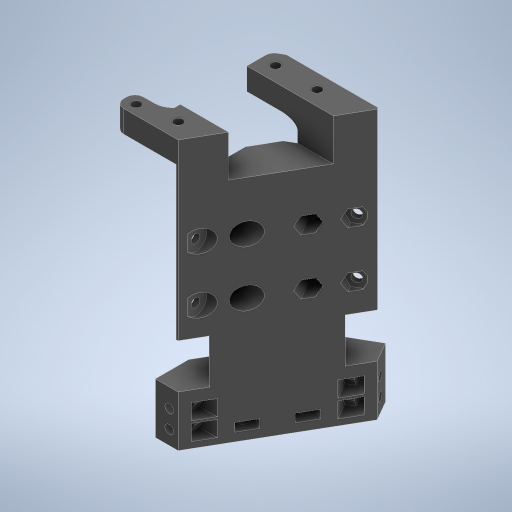
# Autodesk Inventor part: base_plate_towheel_front_right
Saved by Autodesk Inventor 2024.1 (Build 281209000, 209)
## iProperties
Created: 2025-02-03
Part Number: base_plate_towheel_front_right
Material: 一般
Document SubType Name: モデリング
Designer: hibik
Density: 1 g/cm^3
Appearance: 既定
Sheet Metal Rule: Default_mm
Author: hibik
Autodesk Inventor part; units mm, degrees
ref_plane "YZ Plane" through (0, 0, 0) normal (1, 0, 0) x (0, 1, 0)
ref_plane "XZ Plane" through (0, 0, 0) normal (0, 1, 0) x (-1, 0, 0)
ref_plane "XY Plane" through (0, 0, 0) normal (0, 0, 1) x (1, 0, 0)
sketch "スケッチ1" plane through (0, 0, 0) normal (0, 1, 0) x (-1, 0, 0)
  line L0 (75, 0) -> (105, -51.9615)
  line L1 (-75, 0) -> (-105, -51.9615)
  line L2 (0, -220.136) -> (0, 47.7586) projected
  line L3 (147, 0) -> (-147, 0) projected
  line L4 (37.5, -27) -> (-37.5, -27)
  line L5 (105, -51.9615) -> (30, -181.8653)
  line L6 (30, -181.8653) -> (-30, -181.8653)
  line L7 (-30, -181.8653) -> (-105, -51.9615)
  line L8 (75, 0) -> (-75, 0)
  line L9 (-25.3673, -135.8894) -> (-62.8673, -70.9375)
  line L10 (25.3673, -135.8894) -> (62.8673, -70.9375)
  line L11 (-37.5, -27) -> (-27.5, -27)
  line L12 (-27.5, -27) -> (-27.5, -39)
  line L13 (-27.5, -39) -> (-37.5, -39)
  line L14 (-37.5, -39) -> (-37.5, -27)
  line L15 (37.5, -27) -> (27.5, -27)
  line L16 (27.5, -27) -> (27.5, -39)
  line L17 (27.5, -39) -> (37.5, -39)
  line L18 (37.5, -39) -> (37.5, -27)
  line L19 (0, -77.9423) -> (44.1173, -103.4134) construction
  line L20 (0, -77.9423) -> (-44.1173, -103.4134) construction
  line L21 (-44.1173, -103.4134) -> (-67.5, -116.9134) construction
  line L22 (-57.8673, -79.5977) -> (-47.475, -73.5977)
  line L23 (-52.475, -64.9375) -> (-62.8673, -70.9375)
  line L24 (-62.8673, -70.9375) -> (-57.8673, -79.5977)
  line L25 (-47.475, -73.5977) -> (-52.475, -64.9375)
  line L26 (-25.3673, -135.8894) -> (-30.3673, -127.2291)
  line L27 (-19.975, -121.2291) -> (-14.975, -129.8894)
  line L28 (-14.975, -129.8894) -> (-25.3673, -135.8894)
  line L29 (-30.3673, -127.2291) -> (-19.975, -121.2291)
  line L30 (30.3673, -127.2291) -> (19.975, -121.2291)
  line L31 (14.975, -129.8894) -> (25.3673, -135.8894)
  line L32 (25.3673, -135.8894) -> (30.3673, -127.2291)
  line L33 (19.975, -121.2291) -> (14.975, -129.8894)
  line L34 (62.8673, -70.9375) -> (57.8673, -79.5977)
  line L35 (47.475, -73.5977) -> (52.475, -64.9375)
  line L36 (52.475, -64.9375) -> (62.8673, -70.9375)
  line L37 (57.8673, -79.5977) -> (47.475, -73.5977)
  line L38 (62.8673, -70.9375) -> (37.5, -27)
  line L39 (-37.5, -27) -> (-62.8673, -70.9375)
  line L40 (-25.3673, -135.8894) -> (25.3673, -135.8894)
  line L41 (-27.5, -39) -> (-47.475, -73.5977)
  point P0 (0, 0)
  point P1 (0, 0)
  point P2 (0, -27)
  dimension "d1" = 150
  dimension "d2" = 60
  dimension "d3" = 60
  dimension "d4" = 27
  dimension "d5" = 75
  dimension "d6" = 60
  dimension "d7" = 27
  dimension "d8" = 10
  dimension "d9" = 12
  dimension "d10" = 10
  dimension "d11" = 12
  dimension "d14" = 360
  constraints: 80 end point, 6 equal length, 6 parallel, 4 horizontal, 4 midpoint, 3 coincident, 3 perpendicular, 2 symmetric about line, 1 collinear, 1 horizontal alignment, 1 point on line, 1 vertical alignment, 50 other
  measures "d1" distance of L1.start L0.start
  measures "d2" angle of L3 L0
  measures "d3" angle of L1 L3
  measures "d4" distance between parallel lines of L3 L4
  measures "d5" distance of L4.start L4.end
  measures "d6" distance of L5.end L6.end
  measures "d7" distance between parallel lines of L7 L9
  measures "d8" distance of L12.end L13.end
  measures "d9" distance of L11.end L12.end
  measures "d10" distance of L17.end L16.end
  measures "d11" distance of L16.end L15.end
extrude "押し出し1" add sketch "スケッチ1" along normal blind 18.3 contours L12 L13 L14 L4 | L14 L13 L41 L25 L23 L39 | L23 L25 L22 L9
sketch "スケッチ2" plane through (27.5, 0, -27) normal (0, 0, 1) x (1, 0, 0)
  circle A0 centre (5, 11.5) radius 1.6 projected
  circle A1 centre (5, 5) radius 1.6 projected
  point P0 (-27.5, 0)
sketch "スケッチ3" plane through (27.5, 0, -27) normal (0, 0, 1) x (1, 0, 0)
  circle A0 centre (5, 11.5) radius 1.6 projected
  circle A1 centre (5, 5) radius 1.6 projected
  line L0 (8.2909, 11.5) -> (6.6454, 8.65)
  line L1 (6.6454, 8.65) -> (3.3546, 8.65)
  line L2 (3.3546, 8.65) -> (1.7091, 11.5)
  line L3 (1.7091, 11.5) -> (3.3546, 14.35)
  line L4 (3.3546, 14.35) -> (6.6454, 14.35)
  line L5 (6.6454, 14.35) -> (8.2909, 11.5)
  line L6 (6.6454, 7.85) -> (8.2909, 5)
  line L7 (8.2909, 5) -> (6.6454, 2.15)
  line L8 (6.6454, 2.15) -> (3.3546, 2.15)
  line L9 (3.3546, 2.15) -> (1.7091, 5)
  line L10 (1.7091, 5) -> (3.3546, 7.85)
  line L11 (3.3546, 7.85) -> (6.6454, 7.85)
  point P0 (-27.5, 0)
  dimension "d19" = 5.7
  constraints: 24 end point, 2 coincident, 2 horizontal, 1 parallel, 26 other
  measures "d19" distance from line of L0.end L4
extrude "押し出し2" cut sketch "スケッチ3" against normal blind 6 contours A0 | A1 | L0 L1 L2 L3 L4 L5 | L6 L7 L8 L9 L10 L11
extrude "押し出し3" add sketch "スケッチ3" against normal blind 3
sketch "スケッチ4" plane through (27.5, 0, -33) normal (0, 0, 1) x (1, 0, 0)
  line L0 (3.3546, 14.35) -> (6.6454, 14.35)
  line L1 (1.7091, 11.5) -> (3.3546, 14.35)
  line L2 (3.3546, 8.65) -> (1.7091, 11.5)
  line L3 (6.6454, 8.65) -> (3.3546, 8.65)
  line L4 (1.7091, 5) -> (3.3546, 7.85)
  line L5 (3.3546, 2.15) -> (1.7091, 5)
  line L6 (6.6454, 2.15) -> (3.3546, 2.15)
  line L7 (3.3546, 7.85) -> (6.6454, 7.85)
  line L8 (3.3546, 14.35) -> (6.6454, 14.35) projected
  line L9 (6.6454, 14.35) -> (42.8044, 14.35)
  line L10 (42.8044, 14.35) -> (42.8044, 8.65)
  line L11 (42.8044, 8.65) -> (6.6454, 8.65)
  line L12 (6.6454, 7.85) -> (42.8044, 7.85)
  line L13 (42.8044, 7.85) -> (42.8044, 2.15)
  line L14 (42.8044, 2.15) -> (6.6454, 2.15)
  line L15 (6.6454, 14.35) -> (3.3546, 14.35) projected
  line L16 (3.3546, 14.35) -> (1.7091, 11.5) projected
  line L17 (1.7091, 11.5) -> (3.3546, 8.65) projected
  line L18 (3.3546, 8.65) -> (6.6454, 8.65) projected
  line L19 (3.3546, 7.85) -> (1.7091, 5) projected
  line L20 (6.6454, 7.85) -> (3.3546, 7.85) projected
  line L21 (8.2909, 5) -> (6.6454, 7.85) projected
  line L22 (6.6454, 2.15) -> (8.2909, 5) projected
  line L23 (3.3546, 2.15) -> (6.6454, 2.15) projected
  line L24 (1.7091, 5) -> (3.3546, 2.15) projected
  circle A0 centre (5, 5) radius 1.6 projected
  line L25 (6.6454, 7.85) -> (3.3546, 7.85) projected
  line L26 (3.3546, 7.85) -> (1.7091, 5) projected
  line L27 (1.7091, 5) -> (3.3546, 2.15) projected
  line L28 (3.3546, 2.15) -> (6.6454, 2.15) projected
  point P0 (-27.5, 0)
  constraints: 28 end point, 2 horizontal, 2 parallel, 2 perpendicular, 2 point on line, 1 collinear
extrude "押し出し4" cut sketch "スケッチ4" along normal blind 3 contours L0 L9 L10 L11 L3 L2 L1 | L4 L7 L21 L22 L6 L5 | L12 L13 L14 L22 L21 | A0
sketch "スケッチ5" plane through (62.8673, 0, -70.9375) normal (0.8660254, 0, 0.5) x (0.5, 0, -0.8660254)
  line L0 (-5.3923, 18.3) -> (-45.3423, 18.3) projected
  line L1 (-25.3673, 18.3) -> (-25.3673, 0)
  line L2 (-5.3923, 0) -> (-45.3423, 0) projected
  point P0 (-92.8673, 0)
  constraints: 2 end point, 2 midpoint
ref_plane "作業平面1" through (50.1837, 18.3, -48.9687) normal (-0.5, 0, 0.8660254) x (0, -1, 0)
mirror "ミラー1" about plane through (50.1837, 18.3, -48.9687) normal (-0.5, 0, 0.8660254) of "押し出し2", "押し出し3", "押し出し4"
sketch "スケッチ6" plane through (0, 0, 0) normal (0, -1, 0) x (1, 0, 0)
  line L0 (37.5, -27) -> (62.8673, -70.9375) projected
  circle A0 centre (40.9875, -45.0405) radius 1.6
  line L1 (42.7196, -48.0405) -> (39.2555, -48.0405)
  line L2 (39.2555, -48.0405) -> (37.5234, -45.0405)
  line L3 (37.5234, -45.0405) -> (39.2555, -42.0405)
  line L4 (39.2555, -42.0405) -> (42.7196, -42.0405)
  line L5 (42.7196, -42.0405) -> (44.4516, -45.0405)
  line L6 (44.4516, -45.0405) -> (42.7196, -48.0405)
  line L7 (50.1837, -48.9687) -> (37.4875, -56.2989)
  line L8 (47.475, -73.5977) -> (27.5, -39) projected
  line L9 (37.6966, -45.0405) -> (39.3421, -42.1905)
  line L10 (39.3421, -42.1905) -> (42.633, -42.1905)
  line L11 (42.633, -42.1905) -> (44.2784, -45.0405)
  line L12 (44.2784, -45.0405) -> (42.633, -47.8905)
  line L13 (42.633, -47.8905) -> (39.3421, -47.8905)
  line L14 (39.3421, -47.8905) -> (37.6966, -45.0405)
  point P0 (0, 0)
  dimension "d27" = 3.2
  dimension "d29" = 6
  dimension "d30" = 6
  dimension "d31" = 8
  dimension "d32" = 5.7
  constraints: 26 end point, 2 coincident, 2 midpoint, 2 parallel, 1 centre point, 26 other
  measures "d27" diameter of A0
  measures "d29" distance between parallel lines of L2 L5
  measures "d30" distance from line of L0 A0.centre
  measures "d31" distance from line of L7 A0.centre
  measures "d32" distance between parallel lines of L14 L11
extrude "押し出し5" cut sketch "スケッチ6" against normal through all contours A0 | L9 L10 L11 L12 L13 L14
extrude "押し出し7" add sketch "スケッチ6" against normal blind 3 contours L9 L10 L11 L12 L13 L14
mirror "ミラー2" about plane through (50.1837, 18.3, -48.9687) normal (-0.5, 0, 0.8660254) of "押し出し5", "押し出し7"
sketch "スケッチ10" plane through (0, 0, 0) normal (0, -1, 0) x (1, 0, 0)
  line L0 (75, 0) -> (105, -51.9615)
  line L1 (75, 0) -> (81.3804, 3.6837)
  line L2 (37.5, -27) -> (62.8673, -70.9375) projected
  line L3 (50.1837, -48.9687) -> (90, -25.9808)
  line L4 (-21, 0) -> (126, 0) projected
  line L5 (75, 0) -> (35, 0)
  line L6 (45, 0) -> (45, -18)
  line L7 (45, -18) -> (35, -23.7735)
  line L8 (35, 0) -> (35, -23.7735)
  line L9 (35, -23.7735) -> (49.7058, -49.2446)
  line L10 (105, -51.9615) -> (75, 0)
  line L11 (85, -86.6025) -> (64.4115, -74.7158)
  line L12 (64.4115, -74.7158) -> (49.7058, -49.2446)
  line L13 (85, -86.6025) -> (105, -51.9615)
  line L14 (62.8673, -70.9375) -> (57.8673, -79.5977) projected
  line L15 (61.9714, -72.4893) -> (35.6987, -26.9836)
  line L16 (27.5, -27) -> (37.5, -27) projected
  point P0 (0, 0)
  point P1 (35.7081, -27)
  dimension "d47" = 60
  dimension "d48" = 40
  dimension "d49" = 18
  dimension "d50" = 30
  dimension "d51" = 60
  dimension "d63" = 1
  constraints: 28 end point, 5 perpendicular, 5 point on line, 4 symmetric about line, 2 midpoint, 2 parallel
  measures "d47" distance from line of L0.end L1
  measures "d48" distance of L5.end L0.start
  measures "d49" distance of L6.start L6.end
  measures "d50" distance of L0.start L6.start
  measures "d51" angle of L6 L7
  measures "d63" distance between parallel lines of L12 L15
sketch "スケッチ8" plane through (0, 18.3, 0) normal (0, 1, 0) x (1, 0, 0)
  line L0 (47.475, 73.5977) -> (27.5, 39) projected
  line L1 (47.3421, 61.7469) -> (50.633, 61.7469) projected
  line L2 (50.633, 61.7469) -> (52.2784, 58.8969) projected
  line L3 (52.2784, 58.8969) -> (50.633, 56.0469) projected
  line L4 (50.633, 56.0469) -> (47.3421, 56.0469) projected
  line L5 (47.3421, 56.0469) -> (45.6966, 58.8969) projected
  line L6 (45.6966, 58.8969) -> (47.3421, 61.7469) projected
  line L7 (42.633, 47.8905) -> (44.2784, 45.0405) projected
  line L8 (44.2784, 45.0405) -> (42.633, 42.1905) projected
  line L9 (42.633, 42.1905) -> (39.3421, 42.1905) projected
  line L10 (39.3421, 42.1905) -> (37.6966, 45.0405) projected
  line L11 (37.6966, 45.0405) -> (39.3421, 47.8905) projected
  line L12 (39.3421, 47.8905) -> (42.633, 47.8905) projected
  line L13 (57.8673, 79.5977) -> (47.475, 73.5977) projected
  line L14 (47.475, 73.5977) -> (27.5, 39) projected
  line L15 (27.5, 39) -> (27.5, 27) projected
  line L16 (27.5, 27) -> (37.5, 27) projected
  line L17 (37.5, 27) -> (62.8673, 70.9375) projected
  line L18 (62.8673, 70.9375) -> (57.8673, 79.5977) projected
  line L19 (42.633, 47.8905) -> (47.8291, 44.8905)
  line L20 (39.3421, 42.1905) -> (44.5382, 39.1905)
  line L21 (47.3421, 56.0469) -> (52.5382, 53.0469)
  line L22 (50.633, 61.7469) -> (55.8291, 58.7469)
  line L23 (37.5, 27) -> (62.8673, 70.9375) projected
  point P0 (0, 0)
  constraints: 8 end point, 4 perpendicular, 4 point on line
extrude "押し出し9" cut sketch "スケッチ8" against normal up to surface (15.3 mm away) contours L17 L21 L4 L3 L2 L22 | L20 L9 L8 L7 L19 L17
sketch "スケッチ11" plane through (0, 18.3, 0) normal (0, 1, 0) x (1, 0, 0)
  line L0 (52.5382, 53.0469) -> (47.3421, 56.0469) projected
  line L1 (47.3421, 56.0469) -> (45.6966, 58.8969) projected
  line L2 (45.6966, 58.8969) -> (47.3421, 61.7469) projected
  line L3 (47.3421, 61.7469) -> (50.633, 61.7469) projected
  line L4 (50.633, 61.7469) -> (55.8291, 58.7469) projected
  line L5 (55.8291, 58.7469) -> (62.8673, 70.9375) projected
  line L6 (62.8673, 70.9375) -> (57.8673, 79.5977) projected
  line L7 (57.8673, 79.5977) -> (47.475, 73.5977) projected
  line L8 (47.475, 73.5977) -> (27.5, 39) projected
  line L9 (27.5, 39) -> (27.5, 27) projected
  line L10 (27.5, 27) -> (37.5, 27) projected
  line L11 (37.5, 27) -> (44.5382, 39.1905) projected
  line L12 (44.5382, 39.1905) -> (39.3421, 42.1905) projected
  line L13 (39.3421, 42.1905) -> (37.6966, 45.0405) projected
  line L14 (37.6966, 45.0405) -> (39.3421, 47.8905) projected
  line L15 (39.3421, 47.8905) -> (42.633, 47.8905) projected
  line L16 (42.633, 47.8905) -> (47.8291, 44.8905) projected
  line L17 (47.8291, 44.8905) -> (52.5382, 53.0469) projected
  line L18 (38.5, 27) -> (38.5, 38)
  line L19 (38.5, 38) -> (29.817, 43.0131)
  line L20 (27.5, 27) -> (37.5, 27) projected
  line L21 (47.475, 73.5977) -> (27.5, 39) projected
  line L22 (50.1837, 48.9687) -> (37.4875, 56.2989)
  line L23 (63.3673, 70.0715) -> (53.841, 64.5715)
  line L24 (53.841, 64.5715) -> (45.158, 69.5846)
  line L25 (47.8291, 44.8905) -> (44.5382, 39.1905) projected
  line L26 (55.8291, 58.7469) -> (52.5382, 53.0469) projected
  point P0 (0, 0)
  point P1 (61.8673, 69.2054)
  point P2 (38.5, 28.7321)
  dimension "d52" = 1
  dimension "d53" = 11
  constraints: 10 end point, 3 perpendicular, 3 symmetric about line, 2 midpoint, 2 point on line
  measures "d52" distance from line of L10.end L18
  measures "d53" distance of L18.start L18.end
extrude "押し出し11" add sketch "スケッチ11" along normal blind 78.7 contours L17 L22 L8 L24 L23 L5 L4 L3 L2 L1 L0 | L0 L1 L2 L3 L4 L26 | L17 L16 L15 L14 L13 L12 L11 L18 L19 L8 L22 | L25 L12 L13 L14 L15 L16
fillet "フィレット1" radius 2 2 edges at (38.5, 57.65, -28.7321) (61.8673, 57.65, -69.2054)
sketch "スケッチ13" plane through (0, 97, 0) normal (0, 1, 0) x (1, 0, 0)
  line L0 (85, 86.6025) -> (64.4115, 74.7158) projected
  line L1 (35, 0) -> (35, 23.7735) projected
  arc A0 (58.1353, 62.7413) -> (55.4032, 65.4734) centre (56.4032, 63.7413) ccw projected
  line L2 (55.4032, 65.4734) -> (53.841, 64.5715) projected
  line L3 (53.841, 64.5715) -> (45.158, 69.5846) projected
  line L4 (45.158, 69.5846) -> (29.817, 43.0131) projected
  line L5 (29.817, 43.0131) -> (38.5, 38) projected
  line L6 (38.5, 38) -> (38.5, 36.1962) projected
  arc A1 (38.5, 36.1962) -> (42.2321, 35.1962) centre (40.5, 36.1962) ccw projected
  line L7 (35, 23.7735) -> (35, 57.735)
  line L8 (35, 57.735) -> (64.4115, 74.7158)
  line L9 (38.5, 38) -> (29.817, 43.0131) projected
  line L10 (29.817, 43.0131) -> (27.5, 39) projected
  line L11 (27.5, 39) -> (27.5, 27) projected
  line L12 (27.5, 27) -> (37.5, 27) projected
  line L13 (37.5, 27) -> (42.2321, 35.1962) projected
  arc A2 (38.5, 36.1962) -> (42.2321, 35.1962) centre (40.5, 36.1962) ccw projected
  line L14 (38.5, 36.1962) -> (38.5, 38) projected
  line L15 (45.158, 69.5846) -> (53.841, 64.5715) projected
  line L16 (53.841, 64.5715) -> (55.4032, 65.4734) projected
  arc A3 (58.1353, 62.7413) -> (55.4032, 65.4734) centre (56.4032, 63.7413) ccw projected
  line L17 (58.1353, 62.7413) -> (62.8673, 70.9375) projected
  line L18 (62.8673, 70.9375) -> (57.8673, 79.5977) projected
  line L19 (57.8673, 79.5977) -> (47.475, 73.5977) projected
  line L20 (47.475, 73.5977) -> (45.158, 69.5846) projected
  line L21 (42.2321, 35.1962) -> (58.1353, 62.7413) projected
  point P0 (0, 0)
  point P1 (61.6173, 73.1025)
  point P2 (50.341, 66.5922)
  point P3 (39.975, 60.6073)
  point P4 (35, 51.9904)
  point P5 (35, 27)
  point P6 (35, 40.0207)
  constraints: 4 end point, 1 collinear, 1 vertical
extrude "押し出し13" add sketch "スケッチ13" against normal blind 62.7 contours A0 L2 L3 L8 L18 L17 | L13 L12 L7 L5 L6 A1 | L4 L7 L8
extrude "押し出し14" cut sketch "スケッチ13" against normal up to surface (78.7 mm away) contours L8 L4 L3 | L5 L4 L7
extrude "押し出し15" cut sketch "スケッチ10" against normal through all contours L2 L14 L12 L9 L16 | L9 L12 L14 L15 L16
sketch "スケッチ14" plane through (0, 97, 0) normal (0, 1, 0) x (1, 0, 0)
  circle A0 centre (75, 50.5) radius 8.0371 projected
  circle A1 centre (75, 50.5) radius 12
  line L0 (75, 62.5) -> (35, 62.5)
  line L1 (35, 62.5) -> (35, 38.5)
  line L2 (35, 38.5) -> (75, 38.5)
  line L3 (75, 38.5) -> (75, 62.5)
  line L4 (35, 57.735) -> (35, 27) projected
  point P0 (0, 0)
  dimension "d66" = 24
  constraints: 8 end point, 3 horizontal, 2 parallel, 1 coincident, 1 collinear, 1 perpendicular, 3 other
extrude "押し出し16" cut sketch "スケッチ14" against normal blind 15 contours A1 L2 L1 L0
sketch "スケッチ15" plane through (61.6173, 34.3, -73.1025) normal (-0.5, 0, -0.8660254) x (-0.8660254, 0, 0.5)
  circle A0 centre (5, 10) radius 1.6
  circle A1 centre (15.735, 10) radius 1.6
  line L0 (0, 62.7) -> (0, 0) projected
  line L1 (30.735, 47.7) -> (30.735, 0) projected
  line L2 (13.0207, 0) -> (0, 0) projected
  circle A2 centre (15.735, 30) radius 1.6
  circle A3 centre (5, 30) radius 1.6
  circle A4 centre (15.735, 50) radius 1.6
  circle A5 centre (5, 50) radius 1.6
  point P0 (89.9134, -34.3)
  dimension "d69" = 3.2
  dimension "d71" = 5
  dimension "d72" = 15
  dimension "d73" = 10
  dimension "d76" = 20
  constraints: 6 centre point, 1 equal radius, 1 horizontal alignment, 1 vertical, 8 other
  measures "d69" diameter of A0
  measures "d71" distance from line of L0 A0.centre
  measures "d72" distance from line of L1 A1.centre
  measures "d73" distance from line of L2 A0.centre
  measures "d76" distance of A1.centre A2.centre
extrude "押し出し17" cut sketch "スケッチ15" against normal through all contours A0 | A1 | A2 | A3
ref_plane "作業平面3" through (71.6173, 34.3, -55.782) normal (-0.5, 0, -0.8660254) x (-0.8660254, 0, 0.5)
sketch "スケッチ17" plane through (71.6173, 34.3, -55.782) normal (-0.5, 0, -0.8660254) x (-0.8660254, 0, 0.5)
  circle A0 centre (5, 10) radius 1.6 projected
  circle A1 centre (15.735, 10) radius 1.6 projected
  circle A2 centre (5, 30) radius 1.6 projected
  circle A3 centre (15.735, 30) radius 1.6 projected
  line L0 (30.735, 47.7) -> (21.2051, 47.7) projected
  line L1 (21.2051, 47.7) -> (21.2051, 62.7) projected
  line L2 (0, 62.7) -> (21.2051, 62.7) projected
  line L3 (0, 62.7) -> (0, 0) projected
  line L4 (13.0207, 0) -> (0, 0) projected
  line L5 (13.0207, -16) -> (13.0207, 0) projected
  line L6 (13.0207, -16) -> (24.9904, -16) projected
  line L7 (24.9904, 0) -> (24.9904, -16) projected
  line L8 (30.735, 0) -> (24.9904, 0) projected
  line L9 (30.735, 47.7) -> (30.735, 0) projected
  line L10 (2.9233, 48.4535) -> (1.2201, 51.4035)
  line L11 (1.2201, 51.4035) -> (2.9233, 54.3535)
  line L12 (2.9233, 54.3535) -> (6.3297, 54.3535)
  line L13 (6.3297, 54.3535) -> (8.0329, 51.4035)
  line L14 (8.0329, 51.4035) -> (6.3297, 48.4535)
  line L15 (6.3297, 48.4535) -> (2.9233, 48.4535)
  line L16 (14.0318, 27.05) -> (12.3287, 30)
  line L17 (12.3287, 30) -> (14.0318, 32.95)
  line L18 (14.0318, 32.95) -> (17.4382, 32.95)
  line L19 (17.4382, 32.95) -> (19.1414, 30)
  line L20 (19.1414, 30) -> (17.4382, 27.05)
  line L21 (17.4382, 27.05) -> (14.0318, 27.05)
  line L22 (3.2968, 27.05) -> (1.5936, 30)
  line L23 (1.5936, 30) -> (3.2968, 32.95)
  line L24 (3.2968, 32.95) -> (6.7032, 32.95)
  line L25 (6.7032, 32.95) -> (8.4064, 30)
  line L26 (8.4064, 30) -> (6.7032, 27.05)
  line L27 (6.7032, 27.05) -> (3.2968, 27.05)
  line L28 (14.0318, 7.05) -> (12.3287, 10)
  line L29 (12.3287, 10) -> (14.0318, 12.95)
  line L30 (14.0318, 12.95) -> (17.4382, 12.95)
  line L31 (17.4382, 12.95) -> (19.1414, 10)
  line L32 (19.1414, 10) -> (17.4382, 7.05)
  line L33 (17.4382, 7.05) -> (14.0318, 7.05)
  line L34 (6.7032, 7.05) -> (3.2968, 7.05)
  line L35 (3.2968, 7.05) -> (1.5936, 10)
  line L36 (1.5936, 10) -> (3.2968, 12.95)
  line L37 (3.2968, 12.95) -> (6.7032, 12.95)
  line L38 (6.7032, 12.95) -> (8.4064, 10)
  line L39 (8.4064, 10) -> (6.7032, 7.05)
  point P0 (89.9134, -34.3)
  point P1 (4.6265, 51.4035)
  point P2 (15.735, 30)
  point P3 (5, 30)
  point P4 (15.735, 10)
  point P5 (5, 10)
  dimension "d84" = 5.9
  constraints: 60 end point, 4 coincident, 4 equal length, 4 horizontal, 1 point on line, 65 other
  measures "d84" distance between parallel lines of L33 L30
extrude "押し出し18" cut sketch "スケッチ17" along normal blind 18 contours A0 | A1 | A2 | A3 | L16 L17 L18 L19 L20 L21 | L22 L23 L24 L25 L26 L27 | L28 L29 L30 L31 L32 L33 | L34 L35 L36 L37 L38 L39
ref_plane "作業平面4" through (35, 97, -57.735) normal (0.5, 0, -0.8660254) x (0, -1, 0)
mirror "ミラー4" about plane through (35, 97, -57.735) normal (0.5, 0, -0.8660254) of "押し出し17", "押し出し18"
sketch "スケッチ20" plane through (0, 97, 0) normal (0, 1, 0) x (1, 0, 0)
  line L0 (42.3476, 38.5) -> (25, 38.5)
  line L1 (25, 38.5) -> (25, 27)
  line L2 (25, 27) -> (42.3476, 27)
  line L3 (42.3476, 27) -> (42.3476, 38.5) construction
  line L4 (61.9714, 62.5) -> (25, 62.5)
  line L5 (25, 62.5) -> (25, 73.1025)
  line L6 (25, 73.1025) -> (61.9714, 73.1025)
  line L7 (61.9714, 73.1025) -> (61.9714, 62.5) construction
  line L8 (42.3476, 38.5) -> (35, 38.5) projected
  line L9 (43.2532, 62.5) -> (56.2041, 62.5) projected
  line L10 (35.7081, 27) -> (42.3476, 38.5) projected
  line L11 (35, 38.5) -> (35, 27) projected
  line L12 (56.2041, 62.5) -> (61.9714, 72.4893) projected
  line L13 (61.9714, 72.4893) -> (61.6173, 73.1025) projected
  point P0 (0, 0)
  dimension "d88" = 25
  constraints: 16 end point, 4 parallel, 4 point on line, 3 collinear, 2 horizontal, 2 perpendicular
  measures "d88" distance from line of L5 point (0, 0)
extrude "押し出し19" add sketch "スケッチ20" against normal blind 8
fillet "フィレット2" radius 3 1 edges at (52.4352, 89, -67.8013)
sketch "スケッチ21" plane through (0, 97, 0) normal (0, 1, 0) x (1, 0, 0)
  circle A0 centre (30, 32.75) radius 1.6
  circle A1 centre (30, 67.8013) radius 1.6
  circle A2 centre (45, 67.8013) radius 1.6
  line L0 (25, 38.5) -> (25, 27) projected
  line L1 (25, 73.1025) -> (25, 62.5) projected
  point P0 (0, 0)
  point P1 (25, 32.75)
  point P2 (25, 67.8013)
  dimension "d92" = 3.2
  dimension "d94" = 5
  dimension "d95" = 15
  constraints: 3 centre point, 3 horizontal alignment, 2 equal radius, 2 midpoint, 1 vertical alignment
  measures "d92" diameter of A0
  measures "d94" distance from line of L0 A0.centre
  measures "d95" distance of A1.centre A2.centre
extrude "押し出し20" cut sketch "スケッチ21" against normal blind 15
ref_plane "作業平面5" through (0, 82, 0) normal (0, 1, 0) x (1, 0, 0)
sketch "スケッチ22" plane through (0, 82, 0) normal (0, 1, 0) x (1, 0, 0)
  circle A0 centre (30, 32.75) radius 1.6 projected
  circle A1 centre (30, 67.8013) radius 1.6 projected
  circle A2 centre (45, 67.8013) radius 1.6 projected
  line L0 (28.3546, 35.6) -> (31.6454, 35.6)
  line L1 (31.6454, 35.6) -> (33.2909, 32.75)
  line L2 (33.2909, 32.75) -> (31.6454, 29.9)
  line L3 (31.6454, 29.9) -> (28.3546, 29.9)
  line L4 (28.3546, 29.9) -> (26.7091, 32.75)
  line L5 (26.7091, 32.75) -> (28.3546, 35.6)
  line L6 (43.3546, 70.6513) -> (46.6454, 70.6513)
  line L7 (46.6454, 70.6513) -> (48.2909, 67.8013)
  line L8 (48.2909, 67.8013) -> (46.6454, 64.9513)
  line L9 (46.6454, 64.9513) -> (43.3546, 64.9513)
  line L10 (43.3546, 64.9513) -> (41.7091, 67.8013)
  line L11 (41.7091, 67.8013) -> (43.3546, 70.6513)
  line L12 (28.3546, 70.6513) -> (31.6454, 70.6513)
  line L13 (31.6454, 70.6513) -> (33.2909, 67.8013)
  line L14 (33.2909, 67.8013) -> (31.6454, 64.9513)
  line L15 (31.6454, 64.9513) -> (28.3546, 64.9513)
  line L16 (28.3546, 64.9513) -> (26.7091, 67.8013)
  line L17 (26.7091, 67.8013) -> (28.3546, 70.6513)
  point P0 (0, 0)
  dimension "d99" = 5.7
  constraints: 36 end point, 4 coincident, 2 equal length, 2 horizontal, 1 horizontal alignment, 39 other
  measures "d99" distance between parallel lines of L0 L3
extrude "押し出し21" cut sketch "スケッチ22" along normal blind 13 contours A2 | L6 L7 L8 L9 L10 L11
ref_plane "作業平面6" through (-35.7518, 33.3, -57.3077) normal (0, 1, 0) x (-1, 0, 0)
sketch "スケッチ23" plane through (-35.7518, 33.3, -57.3077) normal (0, 1, 0) x (-1, 0, 0)
  line L0 (-14.595, 9.2945) -> (-0.7518, 17.2869) projected
  line L1 (-9.8113, 1.0088) -> (-14.595, 9.2945) projected
  line L2 (-0.7518, 5.3173) -> (1.7357, 1.0088) projected
  line L3 (-0.7518, 17.2869) -> (-0.7518, 5.3173) projected
  circle A0 centre (-8.4479, 6.6474) radius 1.6 projected
  line L4 (-70.7518, 5.3173) -> (-75.7268, -3.2997) projected
  line L5 (1.7357, 1.0088) -> (-73.2393, 1.0088)
  line L6 (-35.7518, 1.0088) -> (-35.7518, 13.8519) construction
  line L7 (-56.9085, 9.2945) -> (-70.7518, 17.2869)
  line L8 (-72.2495, -17.2769) -> (-56.9085, 9.2945)
  line L9 (-86.0928, -9.2845) -> (-72.2495, -17.2769)
  line L10 (-75.7268, -3.2997) -> (-86.0928, -9.2845)
  line L11 (-70.7518, 5.3173) -> (-75.7268, -3.2997)
  line L12 (-70.7518, 17.2869) -> (-70.7518, 5.3173)
  circle A1 centre (-73.0306, -10.6298) radius 1.6
  circle A2 centre (-63.0556, 6.6474) radius 1.6
  line L13 (-73.2393, 1.0088) -> (1.7357, 1.0088)
  line L14 (-64.579, -3.9912) -> (-73.2393, 1.0088)
  line L15 (1.7357, 1.0088) -> (-9.8113, 1.0088) projected
  point P0 (-35.7518, 57.3077)
  point P1 (-70.7518, -0.4274)
  point P2 (-73.2393, 1.0088)
  point P3 (-61.6923, 1.0088)
  constraints: 20 end point, 5 symmetric about line, 4 midpoint, 2 centre point, 2 perpendicular, 2 point on line, 1 other
ref_plane "作業平面7" through (-35.7518, 28.3, -57.3077) normal (0, -1, 0) x (1, 0, 0)
sketch "スケッチ24" plane through (-35.7518, 28.3, -57.3077) normal (0, -1, 0) x (1, 0, 0)
  line L0 (10.0934, 9.4974) -> (11.7388, 6.6474) projected
  line L1 (11.7388, 6.6474) -> (10.0934, 3.7974) projected
  line L2 (10.0934, 3.7974) -> (6.8025, 3.7974) projected
  line L3 (6.8025, 3.7974) -> (5.157, 6.6474) projected
  line L4 (5.157, 6.6474) -> (6.8025, 9.4974) projected
  line L5 (6.8025, 9.4974) -> (10.0934, 9.4974) projected
  line L6 (14.595, 9.2945) -> (0.7518, 17.2869) projected
  line L7 (0.7518, 5.3173) -> (0.7518, 17.2869) projected
  line L8 (-1.7357, 1.0088) -> (0.7518, 5.3173) projected
  line L9 (9.8113, 1.0088) -> (14.595, 9.2945) projected
  line L10 (35.7518, 1.0088) -> (35.7518, 13.8519) construction
  line L11 (71.3852, -13.4798) -> (74.6761, -13.4798)
  line L12 (74.6761, -13.4798) -> (76.3215, -10.6298)
  line L13 (76.3215, -10.6298) -> (74.6761, -7.7798)
  line L14 (74.6761, -7.7798) -> (71.3852, -7.7798)
  line L15 (71.3852, -7.7798) -> (69.7397, -10.6298)
  line L16 (69.7397, -10.6298) -> (71.3852, -13.4798)
  line L17 (61.4102, 9.4974) -> (59.7647, 6.6474)
  line L18 (59.7647, 6.6474) -> (61.4102, 3.7974)
  line L19 (61.4102, 3.7974) -> (64.7011, 3.7974)
  line L20 (64.7011, 3.7974) -> (66.3465, 6.6474)
  line L21 (66.3465, 6.6474) -> (64.7011, 9.4974)
  line L22 (64.7011, 9.4974) -> (61.4102, 9.4974)
  line L23 (56.9085, 9.2945) -> (70.7518, 17.2869)
  line L24 (70.7518, 5.3173) -> (70.7518, 17.2869)
  line L25 (75.7268, -3.2997) -> (70.7518, 5.3173)
  line L26 (86.0928, -9.2845) -> (75.7268, -3.2997)
  line L27 (86.0928, -9.2845) -> (72.2495, -17.2769)
  line L28 (72.2495, -17.2769) -> (56.9085, 9.2945)
  line L29 (-1.7357, 1.0088) -> (9.8113, 1.0088) projected
  point P0 (35.7518, 57.3077)
  constraints: 36 end point, 9 symmetric about line
extrude "押し出し22" add sketch "スケッチ23" against normal up to surface (5 mm away) contours L12 L7 L8 L5 L4
extrude "押し出し23" cut sketch "スケッチ24" against normal blind 2 contours L16 L15 L14 L13 L12 L11 | L22 L21 L20 L19 L18 L17
sketch "スケッチ25" plane through (37, 43.1846, -29.2376) normal (1, 0, 0) x (0, 0, -1)
  circle A0 centre (2.7624, 1.1154) radius 1.6 projected
  circle A1 centre (13.4974, 1.1154) radius 1.6 projected
  circle A2 centre (2.7624, 1.1154) radius 4
  circle A3 centre (13.4974, 1.1154) radius 4
  circle A4 centre (2.7624, 21.1154) radius 1.6 projected
  circle A5 centre (13.4974, 21.1154) radius 1.6 projected
  circle A6 centre (2.7624, 21.1154) radius 4
  circle A7 centre (13.4974, 21.1154) radius 4
  point P0 (-29.2376, -43.1846)
  point P1 (1.0592, 4.0654)
  point P2 (15.2006, 4.0654)
  dimension "d108" = 8
  constraints: 4 centre point, 4 coincident, 3 equal radius
  measures "d108" diameter of A2
extrude "押し出し24" cut sketch "スケッチ25" along normal through all contours A0 | A1 | A2 | A3 | A4 | A6 | A7
sketch "スケッチ26" plane through (0, 18.3, 0) normal (0, -1, 0) x (1, 0, 0)
  line L0 (46.4852, -45.6664) -> (43.1943, -39.9664) projected
  line L1 (43.1943, -39.9664) -> (39.3421, -42.1905) projected
  line L2 (39.3421, -42.1905) -> (37.6966, -45.0405) projected
  line L3 (37.6966, -45.0405) -> (39.3421, -47.8905) projected
  line L4 (39.3421, -47.8905) -> (42.633, -47.8905) projected
  line L5 (42.633, -47.8905) -> (46.4852, -45.6664) projected
  line L6 (35, -51.9904) -> (37.4875, -56.2989) projected
  line L7 (54.4852, -59.5228) -> (51.1943, -53.8228) projected
  line L8 (51.1943, -53.8228) -> (47.3421, -56.0469) projected
  line L9 (47.3421, -56.0469) -> (45.6966, -58.8969) projected
  line L10 (45.6966, -58.8969) -> (47.3421, -61.7469) projected
  line L11 (47.3421, -61.7469) -> (50.633, -61.7469) projected
  line L12 (50.633, -61.7469) -> (54.4852, -59.5228) projected
  point P0 (0, 0)
  point P1 (39.975, -60.6073)
extrude "押し出し25" add sketch "スケッチ26" along normal blind 12.3
sketch "スケッチ27" plane through (27.5, 0, -33) normal (0, 0, 1) x (1, 0, 0)
  line L0 (9.9402, 14.35) -> (9.9402, 8.65) projected
  line L1 (3.3546, 8.65) -> (9.9402, 8.65) projected
  line L2 (1.7091, 11.5) -> (3.3546, 8.65) projected
  line L3 (3.3546, 14.35) -> (1.7091, 11.5) projected
  line L4 (9.9402, 14.35) -> (3.3546, 14.35) projected
  circle A0 centre (5, 11.5) radius 1.6 projected
  line L5 (9.9402, 7.85) -> (9.9402, 2.15) projected
  line L6 (3.3546, 2.15) -> (9.9402, 2.15) projected
  line L7 (1.7091, 5) -> (3.3546, 2.15) projected
  line L8 (3.3546, 7.85) -> (1.7091, 5) projected
  line L9 (9.9402, 7.85) -> (3.3546, 7.85) projected
  circle A1 centre (5, 5) radius 1.6 projected
  circle A2 centre (5, 11.5) radius 1.6 projected
  line L10 (3.3546, 14.35) -> (6.6454, 14.35)
  line L11 (6.6454, 14.35) -> (8.2909, 11.5)
  line L12 (8.2909, 11.5) -> (6.6454, 8.65)
  line L13 (6.6454, 8.65) -> (3.3546, 8.65)
  line L14 (3.3546, 8.65) -> (1.7091, 11.5)
  line L15 (1.7091, 11.5) -> (3.3546, 14.35)
  line L16 (3.3546, 7.85) -> (6.6454, 7.85)
  line L17 (6.6454, 7.85) -> (8.2909, 5)
  line L18 (8.2909, 5) -> (6.6454, 2.15)
  line L19 (6.6454, 2.15) -> (3.3546, 2.15)
  line L20 (3.3546, 2.15) -> (1.7091, 5)
  line L21 (1.7091, 5) -> (3.3546, 7.85)
  line L22 (9.9402, 14.35) -> (23.2941, 14.35)
  line L23 (23.2941, 14.35) -> (23.2941, 8.65)
  line L24 (23.2941, 8.65) -> (9.9402, 8.65)
  line L25 (9.9402, 8.65) -> (9.9402, 14.35)
  line L26 (9.9402, 2.15) -> (24.2317, 2.15)
  line L27 (24.2317, 2.15) -> (24.2317, 7.85)
  line L28 (24.2317, 7.85) -> (9.9402, 7.85)
  line L29 (9.9402, 7.85) -> (9.9402, 2.15)
  line L30 (11.6722, 8.65) -> (3.3546, 8.65) projected
  line L31 (11.6722, 7.85) -> (3.3546, 7.85) projected
  point P0 (-27.5, 0)
  point P1 (6.6454, 7.85)
  point P2 (6.6454, 14.35)
  point P3 (6.6454, 8.65)
  constraints: 40 end point, 4 parallel, 2 coincident, 2 collinear, 2 horizontal, 2 perpendicular, 26 other
extrude "押し出し26" cut sketch "スケッチ27" against normal blind 3 contours L22 L23 L24 L0 | L0 L1 L12 L11 L4 | L28 L27 L26 L5 | L5 L6 L18 L17 L9
sketch "スケッチ28" plane through (27.5, 0, -27) normal (0, 0, 1) x (1, 0, 0)
  circle A0 centre (5, 11.5) radius 1.6 projected
  circle A1 centre (5, 5) radius 1.6 projected
  point P0 (-27.5, 0)
extrude "押し出し27" cut sketch "スケッチ28" against normal blind 15
sketch "スケッチ29" plane through (0, 0, 0) normal (0, -1, 0) x (1, 0, 0)
  circle A0 centre (40.9875, -45.0405) radius 1.6 projected
  point P0 (0, 0)
extrude "押し出し28" cut sketch "スケッチ29" against normal blind 15
mirror "ミラー5" about plane through (50.1837, 18.3, -48.9687) normal (-0.5, 0, 0.8660254) of "押し出し26", "押し出し27", "押し出し28"
sketch "スケッチ30" plane through (0, 34.3, 0) normal (0, -1, 0) x (1, 0, 0)
  line L0 (35, -51.9904) -> (35, -57.735) projected
  line L1 (35, -57.735) -> (39.975, -60.6073) projected
  line L2 (35, -51.9904) -> (39.975, -60.6073) projected
  point P0 (0, 0)
extrude "押し出し29" cut sketch "スケッチ30" against normal through all
sketch "スケッチ31" plane through (0, 97, 0) normal (0, 1, 0) x (1, 0, 0)
  arc A0 (26.5, 71.8801) -> (25, 69.282) centre (28, 69.282) ccw projected
  line L0 (74.1519, 99.392) -> (26.5, 71.8801) projected
  line L1 (61.6173, 73.1025) -> (25, 73.1025) projected
  line L2 (25, 73.1025) -> (25, 62.5) projected
  point P0 (0, 0)
  point P1 (28.6173, 73.1025)
extrude "押し出し30" cut sketch "スケッチ31" against normal through all
sketch "スケッチ32" plane through (0, 97, 0) normal (0, 1, 0) x (1, 0, 0)
  circle A0 centre (20, 41) radius 5 projected
  line L0 (25, 27) -> (35.7081, 27) projected
  line L1 (25, 27) -> (13, 27)
  line L2 (13, 27) -> (13, 34.1574)
  line L3 (13, 34.1574) -> (25, 34.1574)
  line L4 (25, 34.1574) -> (25, 27)
  circle A1 centre (20, 41) radius 6.8426
  line L5 (25, 34.1574) -> (25, 38.5)
  circle A2 centre (17, 30.5787) radius 1.6
  point P0 (0, 0)
  point P1 (25, 36.3287)
  point P2 (13, 30.5787)
  point P3 (20, 34.1574)
  dimension "d121" = 12
  dimension "d122" = 3.2
  dimension "d123" = 4
  constraints: 10 end point, 2 coincident, 2 horizontal, 2 midpoint, 2 parallel, 1 centre point, 1 horizontal alignment, 1 perpendicular, 1 vertical, 3 other
  measures "d121" distance of L0.start L1.end
  measures "d122" diameter of A2
  measures "d123" distance from line of L2 A2.centre
extrude "押し出し31" add sketch "スケッチ32" against normal up to surface (8 mm away) contours L1 L2 L3 L4 | L3 A1 L5
fillet "フィレット3" radius 3 2 edges at (13, 93, -27) (13, 93, -34.1574)
equation "\"d3\" = d2"
equation "\"d7\" = d4"
equation "\"BendRadius\" = Thickness"
equation "\"BendReliefWidth\" = Thickness"
equation "\"BendReliefDepth\" = 0.5 * Thickness"
equation "\"CornerReliefSize\" = 4 * Thickness"
equation "\"MinimumRemnant\" = 2 * Thickness"
equation "\"TransitionRadius\" = BendRadius"
equation "\"JacobiRadiusSize\" = BendRadius"
equation "\"GapSize\" = Thickness"
equation "\"Thickness\" = 1.5"
